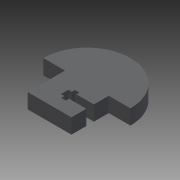
# Autodesk Inventor part: spoolHolder_c
Saved by Autodesk Inventor 2013 (Build 170138000, 138)
## iProperties
Created: 2015-01-14
Part Number: spoolHolder_c
Material: Generic
Document SubType Name: Modeling
Designer: dzban
Density: 1 g/cm^3
Author: dzban
Autodesk Inventor part; units mm, degrees
ref_plane "YZ Plane" through (0, 0, 0) normal (1, 0, 0) x (0, 1, 0)
ref_plane "XZ Plane" through (0, 0, 0) normal (0, 1, 0) x (-1, 0, 0)
ref_plane "XY Plane" through (0, 0, 0) normal (0, 0, 1) x (1, 0, 0)
sketch "Sketch1" plane through (0, 0, 0) normal (0, 0, 1) x (1, 0, 0)
  line L0 (-17.5, 0) -> (-8.8, 0)
  line L1 (-8.8, 0) -> (-8.8, -15)
  line L2 (-8.8, -15) -> (8.8, -15)
  line L3 (8.8, -15) -> (8.8, -9)
  line L4 (8.8, -9) -> (1.8, -9)
  line L5 (1.8, -9) -> (1.8, -10.25)
  line L6 (1.8, -10.25) -> (0, -10.25)
  line L7 (0, -10.25) -> (0, -9)
  line L8 (0, -9) -> (-1.4, -9)
  line L9 (-1.4, -9) -> (-1.4, -6)
  line L10 (-1.4, -6) -> (0, -6)
  line L11 (0, -6) -> (0, -4.75)
  line L12 (0, -4.75) -> (1.8, -4.75)
  line L13 (1.8, -4.75) -> (1.8, -6)
  line L14 (1.8, -6) -> (8.8, -6)
  line L15 (8.8, -6) -> (8.8, 0)
  line L16 (8.8, 0) -> (17.5, 0)
  arc A0 (17.5, 0) -> (-17.5, 0) centre (0, 0) ccw
  point P0 (0, 0)
  constraints: 34 end point, 2 point on circle, 1 centre point
extrude "Extrusion1" add sketch "Sketch1" along normal blind 6
body "Solid1"
